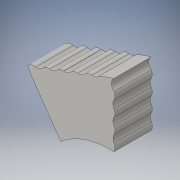
# Autodesk Inventor part: tippa dis claw
Saved by Autodesk Inventor 2016 (Build 200138000, 138)
## iProperties
Created: 2016-01-17
Part Number: tippa dis claw
Material: Generic
Document SubType Name: Modeling
Designer: Josiah Stark
Density: 1 g/cm^3
Appearance: Default
Author: Josiah Stark
Autodesk Inventor part; units mm, degrees
ref_plane "YZ Plane" through (0, 0, 0) normal (1, 0, 0) x (0, 1, 0)
ref_plane "XZ Plane" through (0, 0, 0) normal (0, 1, 0) x (-1, 0, 0)
ref_plane "XY Plane" through (0, 0, 0) normal (0, 0, 1) x (1, 0, 0)
sketch "Sketch1" plane through (0, 0, 0) normal (0, 0, 1) x (1, 0, 0)
  line L0 (0, 0) -> (-1.6764, 0)
  line L1 (-2.8195, 0) -> (-2.8195, -0.0085)
  arc A0 (-2.8195, -0.0085) -> (-18.0949, -6.0198) centre (-1.6549, -25.3818) ccw
  line L2 (-28.1765, 8.5246) -> (-18.0949, -6.0198)
  line L3 (-28.1765, 8.5246) -> (-29.3649, 10.6117)
  line L4 (-17.1011, 15.221) -> (-17.0941, 15.2016)
  line L5 (-9.9296, 17.7969) -> (-9.9234, 17.7799)
  line L6 (-7.5786, 18.7636) -> (-7.5777, 18.7612)
  line L7 (-2.8195, -0.0085) -> (0, 0)
  line L8 (-0.0077, 2.54) -> (0, 0)
  arc A1 (-26.6104, 11.642) -> (-29.3649, 10.6117) centre (-27.262, 9.187) ccw
  arc A2 (-26.6104, 11.642) -> (-24.2313, 12.5319) centre (-26.1915, 14.1472) ccw
  arc A3 (-21.8523, 13.4218) -> (-24.2313, 12.5319) centre (-22.2712, 10.9166) ccw
  arc A4 (-21.8523, 13.4218) -> (-19.4732, 14.3117) centre (-21.4333, 15.927) ccw
  arc A5 (-17.1011, 15.221) -> (-19.4732, 14.3117) centre (-17.4998, 12.7125) ccw
  arc A6 (-17.1011, 15.221) -> (-14.715, 16.0915) centre (-16.6619, 17.7227) ccw
  arc A7 (-12.3359, 16.9814) -> (-14.715, 16.0915) centre (-12.7548, 14.4762) ccw
  arc A8 (-12.3359, 16.9814) -> (-9.9568, 17.8713) centre (-11.917, 19.4866) ccw
  arc A9 (-7.5786, 18.7636) -> (-9.9568, 17.8713) centre (-7.9949, 16.258) ccw
  arc A10 (-7.5786, 18.7636) -> (-5.1986, 19.6511) centre (-7.1571, 21.2684) ccw
  arc A11 (-0.065, 21.5463) -> (-5.1986, 19.6511) centre (6.1141, -3.0906) ccw
  arc A12 (-0.065, 21.5463) -> (-0.0536, 17.7799) centre (1.6451, 19.6683) ccw
  arc A13 (-0.046, 15.2399) -> (-0.0536, 17.7799) centre (-2.2495, 16.5033) ccw
  arc A14 (-0.046, 15.2399) -> (-0.0383, 12.6999) centre (2.1575, 13.9766) ccw
  arc A15 (-0.0307, 10.16) -> (-0.0383, 12.6999) centre (-2.2342, 11.4233) ccw
  arc A16 (-0.0307, 10.16) -> (-0.023, 7.62) centre (2.1729, 8.8966) ccw
  arc A17 (-0.0153, 5.08) -> (-0.023, 7.62) centre (-2.2189, 6.3433) ccw
  arc A18 (-0.0153, 5.08) -> (-0.0077, 2.54) centre (2.1882, 3.8166) ccw
  arc A19 (0, 0) -> (-0.0077, 2.54) centre (-2.2035, 1.2634) ccw
  line L9 (-0.275, 21.4927) -> (-0.0651, 21.5712)
  line L10 (-7.5777, 18.7612) -> (-7.5734, 18.7628)
  line L11 (-29.3649, 10.6117) -> (-26.6104, 11.642)
  line L12 (-17.0941, 15.2016) -> (-17.0604, 15.2142)
  line L13 (-0.0651, 21.5712) -> (-0.065, 21.5463)
  line L14 (-0.0077, 2.54) -> (0, 0)
  line L15 (-2.8195, 0) -> (-2.8195, 3.7275)
  dimension "d14" = 10.6117
  dimension "d15" = 29.3649
  dimension "d21" = 21.5712
  dimension "d22" = 29.2998
  dimension "d25" = 6.0198
  dimension "d26" = 18.0949
  dimension "d27" = 0
  dimension "d30" = 2.54
  dimension "d40" = 2.54
  dimension "d41" = 2.54
  dimension "d42" = 2.54
  dimension "d43" = 2.54
  dimension "d44" = 2.54
  dimension "d45" = 2.54
  dimension "d46" = 2.54
  dimension "d47" = 2.54
  dimension "d48" = 2.54
  dimension "d49" = 2.54
  dimension "d50" = 25.4
  dimension "d51" = 2.54
  dimension "d52" = 2.54
  dimension "d53" = 2.54
  dimension "d54" = 2.54
  dimension "d55" = 2.54
  dimension "d56" = 2.54
  dimension "d57" = 2.54
  dimension "d58" = 2.54
  constraints: 45 point on circle, 32 end point, 20 centre point, 2 perpendicular, 1 horizontal, 1 point on line
  measures "d14" vertical distance of L3.end L0.start
  measures "d15" horizontal distance of L0.start L3.end
  measures "d21" vertical distance of L0.start L9.end
  measures "d22" horizontal distance of L3.end L9.end
  measures "d25" vertical distance of L0.start L2.end
  measures "d26" horizontal distance of L0.start L2.end
  measures "d27" vertical distance of L0.start L1.start
  measures "d30" distance between parallel lines of L6 L5
  measures "d40" radius of A1
  measures "d41" radius of A2
  measures "d42" radius of A3
  measures "d43" radius of A4
  measures "d44" radius of A5
  measures "d45" radius of A6
  measures "d46" radius of A7
  measures "d47" radius of A8
  measures "d48" radius of A9
  measures "d49" radius of A10
  measures "d50" radius of A11
  measures "d51" radius of A12
  measures "d52" radius of A13
  measures "d53" radius of A14
  measures "d54" radius of A15
  measures "d55" radius of A16
  measures "d56" radius of A17
  measures "d57" radius of A18
  measures "d58" radius of A19
extrude "Extrusion1" add sketch "Sketch1" along normal blind 12.7 contours A0 L2 L3 L11 A2 A3 A4 A5 L4 L12 A6 A7 A8 A9 L6 L10 A10 A11 A12 A13 A14 A15 A16 A17 A18 L8 L7 | L8 A19 | A1 L11
sketch "Sketch2" plane through (-18.0949, -6.0198, 0) normal (-0.8219, -0.5697, 0) x (0, 0, 1)
  line L0 (0, 17.6968) -> (0, 0) projected
  line L1 (12.7, 17.751) -> (0, 17.751)
  line L2 (0, 17.751) -> (0, 0)
  line L3 (0, 0) -> (12.7, 0)
  line L4 (12.7, 0) -> (12.7, 17.751)
  line L5 (12.7, 0.1215) -> (0, 0.1215) projected
  line L6 (12.7, 17.751) -> (6.35, 17.751)
  line L7 (6.35, 17.751) -> (6.35, 0.1215)
  line L8 (6.35, 0.1215) -> (12.7, 0.1215)
  line L9 (12.7, 0.1215) -> (12.7, 17.751)
  circle A0 centre (6.35, 7.7415) radius 3.175
  point P0 (0, -5.3609)
  dimension "d62" = 6.35
  dimension "d63" = 7.62
  constraints: 16 end point, 4 parallel, 2 horizontal, 2 perpendicular, 1 centre point, 1 midpoint, 1 point on line
  measures "d62" diameter of A0
  measures "d63" distance from line of L8 A0.centre
extrude "Extrusion2" cut sketch "Sketch2" against normal blind 19.05 contours A0 L7 | L7 A0
body "Solid1"
